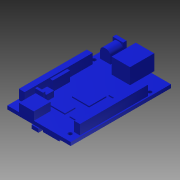
# Autodesk Inventor part: Beagle_Bone_Black
Saved by Autodesk Inventor 2013 (Build 170138000, 138)
## iProperties
Created: 2013-12-19
Material: PC/ABS プラスチック
Document SubType Name: Modeling
Designer: andou
Density: 1.493 g/cm^3
Mass: 42.1596 g
Surface Area: 157.03 cm^2
Volume: 28.2382 cm^3
Author: andou
Title: Beagle_Bone_Black
Autodesk Inventor part; units mm, degrees
ref_plane "YZ Plane" through (0, 0, 0) normal (1, 0, 0) x (0, 1, 0)
ref_plane "XZ Plane" through (0, 0, 0) normal (0, 1, 0) x (-1, 0, 0)
ref_plane "XY Plane" through (0, 0, 0) normal (0, 0, 1) x (1, 0, 0)
sketch "スケッチ1" plane through (0, 0, 0) normal (0, 0, 1) x (1, 0, 0)
  line L0 (-27.5, 43.5) -> (27.5, 43.5)
  line L1 (27.5, 43.5) -> (27.5, -43.5)
  line L2 (27.5, -43.5) -> (-27.5, -43.5)
  line L3 (-27.5, -43.5) -> (-27.5, 43.5)
  point P0 (0, 0)
  dimension "d0" = 87
  dimension "d1" = 55
  dimension "d2" = 27.5
  dimension "d3" = 43.5
  constraints: 8 end point, 2 parallel, 1 horizontal, 1 perpendicular
  measures "d0" distance of L2.end L0.start
  measures "d1" distance of L1.end L2.end
  measures "d2" distance from line of point (0, 0) L3
  measures "d3" distance from line of L2 point (0, 0)
extrude "押し出し1" add sketch "スケッチ1" along normal blind 3
sketch "スケッチ2" plane through (0, 0, 3) normal (0, 0, 1) x (1, 0, 0)
  circle A0 centre (-24.25, 28.5) radius 1.6
  circle A1 centre (24.25, 28.5) radius 1.6
  circle A2 centre (-21, -37.5) radius 1.6
  circle A3 centre (21, -37.5) radius 1.6
  line L0 (-27.5, 43.5) -> (27.5, 43.5) projected
  point P0 (0, 0)
  dimension "d6" = 3.2
  dimension "d7" = 48.5
  dimension "d8" = 42
  dimension "d9" = 21
  dimension "d10" = 24.25
  dimension "d11" = 66
  dimension "d12" = 66
  dimension "d22" = 15
  dimension "d23" = 15
  constraints: 4 centre point, 3 equal radius
  measures "d6" diameter of A1
  measures "d7" distance of A1.centre A0.centre
  measures "d8" distance of A3.centre A2.centre
  measures "d9" horizontal distance of point (0, 0) A2.centre
  measures "d10" horizontal distance of A1.centre point (0, 0)
  measures "d11" vertical distance of A3.centre A1.centre
  measures "d12" vertical distance of A0.centre A2.centre
  measures "d22" distance from line of L0 A0.centre
  measures "d23" distance from line of L0 A1.centre
hole "穴1" at (-21, -37.5, 3) at (21, -37.5, 3) at (24.25, 28.5, 3) at (-24.25, 28.5, 3) direction (0, 0, -1) diameter 3.2 end through all
sketch "スケッチ3" plane through (0, 0, 3) normal (0, 0, 1) x (1, 0, 0)
  line L0 (27.5, -43.5) -> (-27.5, -43.5) projected
  line L1 (-26.5, 24.5) -> (-21.5, 24.5)
  line L2 (-21.5, 24.5) -> (-21.5, -34.5)
  line L3 (-21.5, -34.5) -> (-26.5, -34.5)
  line L4 (-26.5, -34.5) -> (-26.5, 24.5)
  line L5 (21.5, 24.5) -> (26.5, 24.5)
  line L6 (26.5, 24.5) -> (26.5, -34.5)
  line L7 (26.5, -34.5) -> (21.5, -34.5)
  line L8 (21.5, -34.5) -> (21.5, 24.5)
  point P0 (0, 0)
  dimension "d24" = 5
  dimension "d25" = 59
  dimension "d26" = 9
  dimension "d27" = 9
  dimension "d28" = 43
  dimension "d29" = 21.5
  constraints: 16 end point, 4 parallel, 2 equal length, 2 horizontal, 2 perpendicular
  measures "d24" distance of L2.end L3.end
  measures "d25" distance of L3.end L1.start
  measures "d26" distance between parallel lines of L0 L3
  measures "d27" distance between parallel lines of L7 L0
  measures "d28" distance between parallel lines of L8 L2
  measures "d29" distance from line of L8 point (0, 0)
extrude "押し出し2" add sketch "スケッチ3" along normal blind 8.5
sketch "スケッチ4" plane through (0, 0, 3) normal (0, 0, 1) x (1, 0, 0)
  line L0 (-5.5, 25) -> (10.5, 25)
  line L1 (10.5, 25) -> (10.5, 46)
  line L2 (10.5, 46) -> (-5.5, 46)
  line L3 (-5.5, 46) -> (-5.5, 25)
  line L4 (27.5, 43.5) -> (27.5, -43.5) projected
  point P0 (0, 0)
  dimension "d57" = 16
  dimension "d58" = 21
  dimension "d59" = 2.5
  dimension "d60" = 17
  constraints: 8 end point, 2 parallel, 1 horizontal, 1 perpendicular
  measures "d57" distance of L1.end L2.end
  measures "d58" distance of L0.end L1.end
  measures "d59" distance from line of L4.start L2
  measures "d60" distance between parallel lines of L4 L1
extrude "押し出し3" add sketch "スケッチ4" along normal blind 13.5
sketch "スケッチ5" plane through (0, 0, 3) normal (0, 0, 1) x (1, 0, 0)
  line L0 (-22.5, 46) -> (-13.5, 46)
  line L1 (-13.5, 46) -> (-13.5, 32)
  line L2 (-13.5, 32) -> (-22.5, 32)
  line L3 (-22.5, 32) -> (-22.5, 46)
  line L4 (-27.5, -43.5) -> (-27.5, 43.5) projected
  point P0 (5.6589, 43.5)
  dimension "d61" = 5
  dimension "d62" = 9
  dimension "d63" = 14
  dimension "d64" = 2.5
  constraints: 8 end point, 2 parallel, 1 horizontal, 1 perpendicular
  measures "d61" distance between parallel lines of L4 L3
  measures "d62" distance between parallel lines of L3 L1
  measures "d63" distance of L2.end L0.start
  measures "d64" distance from line of L4.end L0
extrude "押し出し4" add sketch "スケッチ5" along normal blind 11
sketch "スケッチ6" plane through (0, 0, 3) normal (0, 0, 1) x (1, 0, 0)
  line L0 (27.5, -43.5) -> (-27.5, -43.5) projected
  line L1 (-17.5, -43.5) -> (-4.5, -43.5)
  line L2 (-4.5, -43.5) -> (-4.5, -29)
  line L3 (-4.5, -29) -> (-17.5, -29)
  line L4 (-17.5, -29) -> (-17.5, -43.5)
  line L5 (-27.5, -43.5) -> (-27.5, 43.5) projected
  point P0 (0, 0)
  dimension "d65" = 13
  dimension "d66" = 10
  dimension "d67" = 14.5
  constraints: 8 end point, 2 parallel, 1 horizontal, 1 perpendicular, 1 point on line
  measures "d65" distance of L2.end L3.end
  measures "d66" distance between parallel lines of L5 L4
  measures "d67" distance between parallel lines of L0 L3
extrude "押し出し5" add sketch "スケッチ6" along normal blind 7
sketch "スケッチ7" plane through (0, 0, 0) normal (0, 0, -1) x (-1, 0, 0)
  line L0 (5.5, -44.5) -> (-0.5, -44.5)
  line L1 (-0.5, -44.5) -> (-0.5, -36.5)
  line L2 (-0.5, -36.5) -> (5.5, -36.5)
  line L3 (5.5, -36.5) -> (5.5, -44.5)
  line L4 (27.5, -43.5) -> (27.5, 43.5) projected
  point P0 (0, 0)
  dimension "d68" = 6
  dimension "d69" = 8
  dimension "d70" = 22
  dimension "d71" = 1
  constraints: 8 end point, 2 parallel, 1 horizontal, 1 perpendicular
  measures "d68" distance of L0.start L0.end
  measures "d69" distance between parallel lines of L0 L2
  measures "d70" distance between parallel lines of L4 L3
  measures "d71" distance from line of L4.start L0
extrude "押し出し6" add sketch "スケッチ7" along normal blind 3
sketch "スケッチ8" plane through (0, 0, 0) normal (0, 0, -1) x (-1, 0, 0)
  line L0 (-27.5, -43.5) -> (-0.5, -43.5) projected
  line L1 (-3.5, -43.5) -> (-17.5, -43.5)
  line L2 (-17.5, -43.5) -> (-17.5, -28.5)
  line L3 (-17.5, -28.5) -> (-3.5, -28.5)
  line L4 (-3.5, -28.5) -> (-3.5, -43.5)
  line L5 (-27.5, 43.5) -> (-27.5, -43.5) projected
  point P0 (0, 0)
  dimension "d72" = 14
  dimension "d73" = 15
  dimension "d74" = 10
  constraints: 8 end point, 2 parallel, 1 horizontal, 1 perpendicular, 1 point on line
  measures "d72" distance of L2.end L3.end
  measures "d73" distance of L1.end L2.end
  measures "d74" distance between parallel lines of L5 L2
extrude "押し出し7" add sketch "スケッチ8" along normal blind 1.5
sketch "スケッチ9" plane through (0, 0, 0) normal (0, 0, -1) x (-1, 0, 0)
  line L0 (-21, 44.5) -> (-13, 44.5)
  line L1 (-13, 44.5) -> (-13, 37.5)
  line L2 (-13, 37.5) -> (-21, 37.5)
  line L3 (-21, 37.5) -> (-21, 44.5)
  line L4 (-27.5, 43.5) -> (-27.5, -43.5) projected
  point P0 (0, 0)
  dimension "d75" = 8
  dimension "d76" = 7
  dimension "d77" = 6.5
  dimension "d78" = 1
  constraints: 8 end point, 2 parallel, 1 horizontal, 1 perpendicular
  measures "d75" distance of L1.end L2.end
  measures "d76" distance of L2.end L0.start
  measures "d77" distance between parallel lines of L4 L3
  measures "d78" distance from line of L4.start L0
extrude "押し出し8" add sketch "スケッチ9" along normal blind 4
sketch "スケッチ11" plane through (0, 0, 3) normal (0, 0, 1) x (1, 0, 0)
  line L0 (-20.5, 1.5) -> (-18, 1.5)
  line L1 (-18, 1.5) -> (-18, -13.5)
  line L2 (-18, -13.5) -> (-20.5, -13.5)
  line L3 (-20.5, -13.5) -> (-20.5, 1.5)
  line L4 (-17.5, -43.5) -> (-27.5, -43.5) projected
  line L5 (-21.5, 24.5) -> (-21.5, -34.5) projected
  point P0 (0, 0)
  dimension "d79" = 15
  dimension "d80" = 2.5
  dimension "d81" = 30
  dimension "d82" = 1
  constraints: 8 end point, 2 parallel, 1 horizontal, 1 perpendicular
  measures "d79" distance of L0.end L1.end
  measures "d80" distance between parallel lines of L3 L1
  measures "d81" distance between parallel lines of L4 L2
  measures "d82" distance between parallel lines of L5 L3
extrude "押し出し10" add sketch "スケッチ11" along normal blind 8.5
sketch "スケッチ12" plane through (0, 0, 3) normal (0, 0, 1) x (1, 0, 0)
  line L0 (-19.5, -17) -> (-13.5, -17)
  line L1 (-13.5, -17) -> (-13.5, -23.5)
  line L2 (-13.5, -23.5) -> (-19.5, -23.5)
  line L3 (-19.5, -23.5) -> (-19.5, -17)
  line L4 (-17.5, -43.5) -> (-27.5, -43.5) projected
  line L5 (-21.5, 24.5) -> (-21.5, -34.5) projected
  point P0 (0, 0)
  dimension "d83" = 6
  dimension "d84" = 6.5
  dimension "d86" = 2
  dimension "d87" = 20
  constraints: 8 end point, 2 parallel, 1 horizontal, 1 perpendicular
  measures "d83" distance of L0.start L0.end
  measures "d84" distance between parallel lines of L0 L2
  measures "d86" distance between parallel lines of L5 L3
  measures "d87" distance between parallel lines of L4 L2
extrude "押し出し11" add sketch "スケッチ12" along normal blind 5
sketch "スケッチ13" plane through (0, 0, 14) normal (0, 0, 1) x (1, 0, 0)
  line L0 (-13.5, 46) -> (-13.5, 32) projected
  line L1 (-22.5, 32) -> (-13.5, 32)
  line L2 (-13.5, 32) -> (-13.5, 43)
  line L3 (-13.5, 43) -> (-22.5, 43)
  line L4 (-22.5, 43) -> (-22.5, 32)
  point P0 (0, 0)
  dimension "d112" = 11
  constraints: 8 end point, 2 parallel, 1 horizontal, 1 perpendicular, 1 point on line
  measures "d112" distance of L3.end L1.start
extrude "押し出し13" cut sketch "スケッチ13" against normal blind 1
sketch "スケッチ14" plane through (0, 0, 3) normal (0, 0, 1) x (1, 0, 0)
  line L0 (-17.5, -43.5) -> (-27.5, -43.5) projected
  line L1 (-21.5, 24.5) -> (-21.5, -34.5) projected
  line L2 (-19.5, -25.5) -> (-12.5, -25.5)
  line L3 (-12.5, -25.5) -> (-12.5, -27.5)
  line L4 (-12.5, -27.5) -> (-19.5, -27.5)
  line L5 (-19.5, -27.5) -> (-19.5, -25.5)
  point P0 (0, 0)
  dimension "d88" = 7
  dimension "d89" = 2
  dimension "d90" = 2
  dimension "d91" = 16
  constraints: 8 end point, 2 parallel, 1 horizontal, 1 perpendicular
  measures "d88" distance of L3.end L4.end
  measures "d89" distance between parallel lines of L2 L4
  measures "d90" distance between parallel lines of L1 L5
  measures "d91" distance between parallel lines of L0 L4
extrude "押し出し14" add sketch "スケッチ14" along normal blind 9
sketch "スケッチ10" plane through (0, 0, 3) normal (0, 0, 1) x (1, 0, 0)
  line L0 (-5.5, 5.5) -> (9.5, 5.5)
  line L1 (9.5, 5.5) -> (9.5, -9.5)
  line L2 (9.5, -9.5) -> (-5.5, -9.5)
  line L3 (-5.5, -9.5) -> (-5.5, 5.5)
  line L4 (-9.5, -16.5) -> (4.5, -16.5)
  line L5 (4.5, -16.5) -> (4.5, -25.5)
  line L6 (4.5, -25.5) -> (-9.5, -25.5)
  line L7 (-9.5, -25.5) -> (-9.5, -16.5)
  line L8 (9.5, 20.5) -> (20.5, 20.5)
  line L9 (20.5, 20.5) -> (20.5, 7.5)
  line L10 (20.5, 7.5) -> (9.5, 7.5)
  line L11 (9.5, 7.5) -> (9.5, 20.5)
  line L12 (27.5, -43.5) -> (-4.5, -43.5) projected
  line L13 (27.5, 43.5) -> (27.5, -43.5) projected
  line L14 (10.5, 43.5) -> (27.5, 43.5) projected
  line L15 (8.5, -16.5) -> (17.5, -16.5)
  line L16 (17.5, -16.5) -> (17.5, -25.5)
  line L17 (17.5, -25.5) -> (8.5, -25.5)
  line L18 (8.5, -25.5) -> (8.5, -16.5)
  point P0 (0, 0)
  dimension "d94" = 11
  dimension "d95" = 15
  dimension "d96" = 14
  dimension "d97" = 9
  dimension "d98" = 9
  dimension "d99" = 9
  dimension "d100" = 15
  dimension "d101" = 13
  dimension "d102" = 23
  dimension "d103" = 38
  dimension "d104" = 18
  dimension "d105" = 18
  dimension "d106" = 7
  dimension "d107" = 18
  dimension "d108" = 10
  dimension "d109" = 4
  constraints: 32 end point, 8 parallel, 4 horizontal, 4 perpendicular
  measures "d94" distance of L8.start L8.end
  measures "d95" distance of L0.start L0.end
  measures "d96" distance of L4.start L4.end
  measures "d97" distance of L16.end L17.end
  measures "d98" distance of L15.end L16.end
  measures "d99" distance of L6.end L4.start
  measures "d100" distance of L2.end L0.start
  measures "d101" distance of L10.end L8.start
  measures "d102" distance between parallel lines of L14 L8
  measures "d103" distance between parallel lines of L14 L0
  measures "d104" distance between parallel lines of L12 L17
  measures "d105" distance between parallel lines of L12 L6
  measures "d106" distance between parallel lines of L13 L9
  measures "d107" distance between parallel lines of L13 L1
  measures "d108" distance between parallel lines of L13 L16
  measures "d109" distance between parallel lines of L18 L5
extrude "押し出し15" add sketch "スケッチ10" along normal blind 1
fillet "フィレット1" radius 4 2 edges at (-13.5, 37.5, 13) (-22.5, 37.5, 13)
